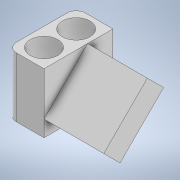
# Autodesk Inventor part: obudowa_stand
Saved by Autodesk Inventor 2020.3 (Build 243373000, 373)
## iProperties
Created: 2021-04-25
Part Number: obudowa_stand
Material: Ogólny
Document SubType Name: Modeling
Designer: patry
Density: 1 g/cm^3
Appearance: Domyślna
Author: patry
Autodesk Inventor part; units mm, degrees
ref_plane "YZ Plane" through (0, 0, 0) normal (1, 0, 0) x (0, 1, 0)
ref_plane "XZ Plane" through (0, 0, 0) normal (0, 1, 0) x (-1, 0, 0)
ref_plane "XY Plane" through (0, 0, 0) normal (0, 0, 1) x (1, 0, 0)
sketch "Szkic1" plane through (0, 0, 0) normal (0, 1, 0) x (-1, 0, 0)
  circle A0 centre (-0.3368, -8.6859) radius 3
  circle A1 centre (-0.3368, -1.6859) radius 3
  line L0 (3.6632, 2.3141) -> (-4.3368, 2.3141)
  line L1 (-4.3368, 2.3141) -> (-4.3368, -12.6859)
  line L2 (-4.3368, -12.6859) -> (3.6632, -12.6859)
  line L3 (3.6632, -12.6859) -> (3.6632, 2.3141)
  point P0 (0, 0)
  dimension "d0" = 6
  dimension "d1" = 6
  dimension "d2" = 7
  dimension "d3" = 8
  dimension "d4" = 15
  dimension "d5" = 4
  dimension "d6" = 4
  constraints: 8 end point, 2 centre point, 2 parallel, 1 horizontal, 1 perpendicular
  measures "d0" diameter of A0
  measures "d1" diameter of A1
  measures "d2" distance of A0.centre A1.centre
  measures "d3" distance of L2.end L1.end
  measures "d4" distance of L1.end L0.end
  measures "d5" distance from line of L3 A1.centre
  measures "d6" distance from line of L0 A1.centre
extrude "Wyciągnięcie proste1" add sketch "Szkic1" along normal blind 13
fillet "Zaokrąglenie1" radius 2 2 edges at (-3.6632, 6.5, 2.3141) (-3.6632, 6.5, -12.6859)
sketch "Szkic2" plane through (4.3368, 0, 0.3141) normal (1, 0, 0) x (0, 0, -1)
  line L0 (6, 13) -> (6, 0) construction
  line L1 (-2, 0) -> (13, 0) projected
  line L2 (13, 0) -> (13, 13) projected
  line L3 (-2, 13) -> (13, 13) projected
  line L4 (-2, 0) -> (-2, 13) projected
  line L5 (-2, 3.5355) -> (1.5355, 0)
  line L6 (-2, 3.5355) -> (3, 3.5355) construction
  line L7 (1.5355, 0) -> (11, 9.4645)
  line L8 (11, 9.4645) -> (7.4645, 13)
  line L9 (7.4645, 13) -> (-2, 3.5355)
  line L10 (-2, 0) -> (-2, 13) construction
  dimension "d18" = 45
  dimension "d19" = 90
  dimension "d20" = 90
  dimension "d21" = 5
  constraints: 10 end point, 5 point on line, 2 equal length, 1 horizontal
  measures "d18" angle of L5 L6
  measures "d19" angle of L7 L5
  measures "d20" angle of L8 L7
  measures "d21" distance of L7.end L8.end
extrude "Wyciągnięcie proste2" add sketch "Szkic2" along normal blind 13 and the other way blind 1 contours L5 L9 L8 L7
